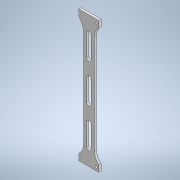
# Autodesk Inventor part: arm_5
Saved by Autodesk Inventor 2020 (Build 240168000, 168)
## iProperties
Created: 2020-01-21
Part Number: arm_5
Material: Generic
Document SubType Name: Modeling
Designer: psrobotics
Density: 1 g/cm^3
Appearance: Default
Author: psrobotics
Autodesk Inventor part; units mm, degrees
ref_plane "YZ Plane" through (0, 0, 0) normal (1, 0, 0) x (0, 1, 0)
ref_plane "XZ Plane" through (0, 0, 0) normal (0, 1, 0) x (-1, 0, 0)
ref_plane "XY Plane" through (0, 0, 0) normal (0, 0, 1) x (1, 0, 0)
sketch "Sketch1" plane through (0, 0, 0) normal (0, 0, 1) x (1, 0, 0)
  line L0 (2.5, -3) -> (-2.5, -3) projected
  line L1 (2.5, 4) -> (2.5, -3) projected
  line L2 (-2.5, 4) -> (2.5, 4) projected
  line L3 (-2.5, -3) -> (-2.5, 4) projected
  circle A0 centre (0, 0.5) radius 1 projected
  line L4 (-10.5, -3) -> (-15.5, -3) projected
  line L5 (-10.5, 4) -> (-10.5, -3) projected
  line L6 (-15.5, 4) -> (-10.5, 4) projected
  line L7 (-15.5, -3) -> (-15.5, 4) projected
  circle A1 centre (-13, 0.5) radius 1 projected
  circle A2 centre (-6.5, -28) radius 1.25 projected
  line L8 (-6.5, -28) -> (-6.5, 142)
  line L9 (-13, 0.5) -> (0, 0.5)
  line L10 (-6.5, 142) -> (-6.5, 113.5)
  line L11 (0, 0.5) -> (0, 113.5)
  line L12 (-13, 0.5) -> (-13, 113.5)
  circle A3 centre (-13, 113.5) radius 1
  circle A4 centre (0, 113.5) radius 1
  line L13 (-15.5, 116.5) -> (2.5, 116.5)
  line L14 (2.5, 116.5) -> (2.5, 110.5)
  line L15 (2.5, 110.5) -> (-15.5, 110.5)
  line L16 (-15.5, 110.5) -> (-15.5, 116.5)
  line L17 (-15.5, 116.5) -> (2.5, 110.5) construction
  line L18 (2.5, 116.5) -> (-15.5, 110.5) construction
  line L19 (-15.5, 3.5) -> (2.5, 3.5)
  line L20 (2.5, 3.5) -> (2.5, -2.5)
  line L21 (2.5, -2.5) -> (-15.5, -2.5)
  line L22 (-15.5, -2.5) -> (-15.5, 3.5)
  line L23 (-15.5, 3.5) -> (2.5, -2.5) construction
  line L24 (2.5, 3.5) -> (-15.5, -2.5) construction
  line L25 (-11.5, 12) -> (-1.5, 12)
  line L26 (-1.5, 12) -> (-1.5, 102)
  line L27 (-1.5, 102) -> (-11.5, 102)
  line L28 (-11.5, 102) -> (-11.5, 12)
  line L29 (-11.5, 12) -> (-1.5, 102) construction
  line L30 (-1.5, 12) -> (-11.5, 102) construction
  arc A5 (-11.5, 102) -> (-15.5, 110.5) centre (-25.9409, 100.3955) ccw
  arc A6 (2.5, 110.5) -> (-1.5, 102) centre (9.5312, 102) ccw
  arc A7 (-15.5, 3.5) -> (-11.5, 12) centre (-22.5313, 12) ccw
  arc A8 (-1.5, 12) -> (2.5, 3.5) centre (9.5313, 12) ccw
  point P0 (0, 0)
  point P1 (-6.5, 0.5)
  point P2 (-6.5, 57)
  point P3 (2.5, -2.5)
  point P4 (2.5, 3.5)
  dimension "d0" = 170
  dimension "d1" = 28.5
  dimension "d2" = 113
  dimension "d3" = 113
  dimension "d4" = 2
  dimension "d5" = 2
  dimension "d6" = 18
  dimension "d7" = 6
  dimension "d8" = 18
  dimension "d9" = 6
  dimension "d10" = 10
  dimension "d11" = 90
  constraints: 46 end point, 8 midpoint, 8 point on circle, 6 centre point, 6 parallel, 5 perpendicular, 3 vertical, 2 coincident, 2 horizontal, 2 line through centre, 2 tangent, 1 point on line
  measures "d0" distance of L8.start L8.end
  measures "d1" distance of L8.end L10.end
  measures "d2" distance of L9.end L11.end
  measures "d3" distance of L9.start L12.end
  measures "d4" diameter of A3
  measures "d5" diameter of A4
  measures "d6" distance of L13.start L13.end
  measures "d7" distance of L13.end L14.end
  measures "d8" distance of L19.start L19.end
  measures "d9" distance of L19.end L20.end
  measures "d10" distance of L25.start L25.end
  measures "d11" distance of L26.end L25.end
extrude "Extrusion1" add sketch "Sketch1" along normal blind 2 contours L21 L3 L9 A0 L11 L19 L1 | L21 L8 L9 L3 | L19 L11 L2 A8 | L9 L8 L19 L3 | L3 L19 L11 A0 L9 | L21 L5 L9 L8 | L19 L3 L2 L11 | L2 L11 A8 | L19 L8 L25 A8 L11 L2 L3 | L9 L5 L19 L8 | L21 L7 L19 L12 A1 L9 L5 | L19 L5 L6 L12 A7 L25 L8 | L9 A1 L12 L19 L5 | A6 L27 L8 L15 L11 | L11 L15 A6 | L25 L8 L27 L26 | L25 L28 L27 L8 | L19 L12 L6 L5 | A7 L6 L12 L19 | L15 L8 L13 L14 | L27 A5 L12 L15 L8 | A7 L12 L6 | L15 L16 L13 L8 | L12 A5 L15
sketch "Sketch2" plane through (0, 0, 2) normal (0, 0, 1) x (1, 0, 0)
  line L0 (-15.5, 3.5) -> (-15.5, -2.5) projected
  line L1 (-15.5, -2.5) -> (2.5, -2.5) projected
  line L2 (2.5, -2.5) -> (2.5, 3.5) projected
  arc A0 (-1.5, 12) -> (2.5, 3.5) centre (9.5313, 12) ccw projected
  line L3 (-1.5, 12) -> (-1.5, 102) projected
  arc A1 (2.5, 110.5) -> (-1.5, 102) centre (9.5312, 102) ccw projected
  line L4 (2.5, 110.5) -> (2.5, 116.5) projected
  line L5 (2.5, 116.5) -> (-15.5, 116.5) projected
  line L6 (-15.5, 116.5) -> (-15.5, 110.5) projected
  arc A2 (-11.5, 102) -> (-15.5, 110.5) centre (-25.9409, 100.3955) ccw projected
  line L7 (-11.5, 102) -> (-11.5, 12) projected
  arc A3 (-15.5, 3.5) -> (-11.5, 12) centre (-22.5313, 12) ccw projected
  circle A4 centre (0, 0.5) radius 1 projected
  circle A5 centre (0, 113.5) radius 1 projected
  circle A6 centre (-13, 113.5) radius 1 projected
  circle A7 centre (-13, 0.5) radius 1 projected
  line L8 (2.5, 116.5) -> (-15.5, 116.5) projected
  line L9 (-6.5, 116.5) -> (-6.5, -2.5)
  line L10 (-6.5, 67) -> (-6.5, 47) construction
  line L11 (-8.5, 67) -> (-8.5, 47)
  line L12 (-4.5, 47) -> (-4.5, 67)
  arc A8 (-4.5, 67) -> (-8.5, 67) centre (-6.5, 67) ccw
  arc A9 (-8.5, 47) -> (-4.5, 47) centre (-6.5, 47) ccw
  line L13 (-6.5, 57) -> (-6.5, 92)
  line L14 (-6.5, 102) -> (-6.5, 82) construction
  line L15 (-8.5, 102) -> (-8.5, 82)
  line L16 (-4.5, 82) -> (-4.5, 102)
  arc A10 (-4.5, 102) -> (-8.5, 102) centre (-6.5, 102) ccw
  arc A11 (-8.5, 82) -> (-4.5, 82) centre (-6.5, 82) ccw
  line L17 (-6.5, 57) -> (-6.5, 22)
  line L18 (-6.5, 32) -> (-6.5, 12) construction
  line L19 (-8.5, 32) -> (-8.5, 12)
  line L20 (-4.5, 12) -> (-4.5, 32)
  arc A12 (-4.5, 32) -> (-8.5, 32) centre (-6.5, 32) ccw
  arc A13 (-8.5, 12) -> (-4.5, 12) centre (-6.5, 12) ccw
  point P0 (0, 0)
  dimension "d14" = 10
  dimension "d15" = 4
  dimension "d16" = 35
  dimension "d17" = 10
  dimension "d18" = 4
  dimension "d19" = 35
  dimension "d20" = 10
  dimension "d21" = 4
  constraints: 30 end point, 12 point on circle, 12 tangent, 6 centre point, 6 midpoint, 5 point on line, 3 parallel
  measures "d14" distance of L13.start L10.end
  measures "d15" diameter of A9
  measures "d16" distance of L13.start L13.end
  measures "d17" distance of L13.end L14.end
  measures "d18" diameter of A11
  measures "d19" distance of L13.start L17.end
  measures "d20" distance of L17.end L18.end
  measures "d21" diameter of A13
extrude "Extrusion2" cut sketch "Sketch2" against normal blind 2 contours A13 L19 A12 L9 | L9 A12 L20 A13 | A9 L11 A8 L9 | L9 A8 L12 A9 | A10 L16 A11 L9 | L9 A11 L15 A10
body "Solid1"
